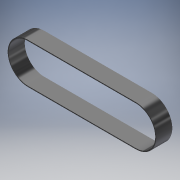
# Autodesk Inventor part: Synchronous Belt1
Saved by Autodesk Inventor 2018 (Build 220112000, 112)
## iProperties
Created: 2018-04-15
Part Number: Synchronous Belt1
Material: Rubber
Document SubType Name: Modeling
Designer: cwsin_000
Density: 0.93 g/cm^3
Appearance: Rubber - Black - Version 1.1
Mass: 5.0592 g
Surface Area: 115.6 cm^2
Volume: 5.44 cm^3
CustomPartVersion: 1
Author: cwsin_000
Autodesk Inventor part; units mm, degrees
sketch "Sketch Path" plane through (0, 0, 0) normal (0, 0, 1) x (1, 0, 0)
  arc A0 (-100, 19.8944) -> (-100, -19.8944) centre (-100, 0) ccw
  arc A1 (7.5, -19.8944) -> (7.5, 19.8944) centre (7.5, 0) ccw
  line L0 (7.5, -19.8944) -> (-100, -19.8944)
  line L1 (-100, 19.8944) -> (7.5, 19.8944)
  constraints: 4 end point, 4 point on circle, 2 centre point
ref_plane "Cross Section Plane" through (-100, -19.8944, 0) normal (1, 0, 0) x (0, 0, 1)
ref_plane "Work Plane2" through (-100, 0, 0) normal (-1, 0, 0) x (0, 0, 1)
ref_plane "Work Plane3" through (7.5, 0, 0) normal (-0.9921, 0.1253, 0) x (0, 0, 1)
sketch "Cross Section" plane through (-100, -19.8944, 0) normal (1, 0, 0) x (0, 0, 1)
  line L0 (-8, 0.5) -> (8, 0.5)
  line L1 (8, 0.5) -> (8, -0.5)
  line L2 (8, -0.5) -> (-8, -0.5)
  line L3 (-8, -0.5) -> (-8, 0.5)
  line L4 (-8, 0) -> (8, 0) construction
  point P0 (0, 0)
  point P1 (0, 0)
  dimension "d0" = 16
  dimension "d4" = 0.5
  dimension "d5" = 0.5
  constraints: 10 end point, 3 midpoint, 2 parallel, 1 coincident, 1 horizontal, 1 perpendicular, 1 other
  measures "d0" distance between parallel lines of L1 L3
  measures "d4" distance between parallel lines of L2 L4
  measures "d5" distance between parallel lines of L4 L0
sweep "Belt" add profiles "Cross Section" path "Sketch Path"
equation "\"d0\" = da_B"
equation "\"d4\" = da_a"
equation "\"d5\" = da_a2"
equation "\"da_B\" = 16"
equation "\"da_pb\" = 5"
equation "\"da_a\" = 0.5"
equation "\"da_S\" = 2.65"
equation "\"da_Beta\" = 20deg"
equation "\"da_Ht\" = 1.2"
equation "\"da_H\" = 2.2"
equation "\"da_a2\" = 0.5"
body "Solid1"
